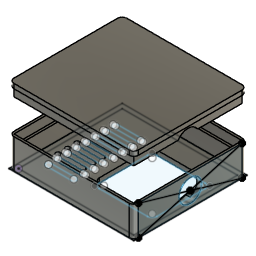
gps&speaker v2 (Autodesk Fusion 360 design; units mm, degrees)
Autodesk Fusion 360 part; units mm, degrees
sketch "Sketch1" plane through (0, 0, 0) normal (0, 0, 1) x (1, 0, 0)
  line L0 (0, 0) -> (50, 0)
  line L1 (50, 0) -> (50, 45)
  line L2 (50, 45) -> (0, 45)
  line L3 (0, 45) -> (0, 0)
  line L4 (-2, -2) -> (52, -2)
  line L5 (52, -2) -> (52, 47)
  line L6 (52, 47) -> (-2, 47)
  line L7 (-2, 47) -> (-2, -2)
  line L8 (25, 35) -> (46, 35)
  line L9 (48, 33) -> (48, 12)
  line L10 (46, 10) -> (25, 10)
  line L11 (23, 12) -> (23, 33)
  arc A0 (25, 35) -> (23, 33) centre (25, 33) ccw
  arc A1 (48, 33) -> (46, 35) centre (46, 33) ccw
  arc A2 (46, 10) -> (48, 12) centre (46, 12) ccw
  arc A3 (23, 12) -> (25, 10) centre (25, 12) ccw
  line L12 (5, 7) -> (16, 7)
  line L13 (16, 9) -> (5, 9)
  arc A4 (4, 8) -> (5, 7) centre (5, 8) ccw
  arc A5 (5, 9) -> (4, 8) centre (5, 8) ccw
  arc A6 (16, 7) -> (17, 8) centre (16, 8) ccw
  arc A7 (17, 8) -> (16, 9) centre (16, 8) ccw
  line L14 (16, 13.1429) -> (5, 13.1429)
  line L15 (5, 11.1429) -> (16, 11.1429)
  arc A8 (4, 12.1429) -> (5, 11.1429) centre (5, 12.1429) ccw
  arc A9 (5, 13.1429) -> (4, 12.1429) centre (5, 12.1429) ccw
  arc A10 (16, 11.1429) -> (17, 12.1429) centre (16, 12.1429) ccw
  arc A11 (17, 12.1429) -> (16, 13.1429) centre (16, 12.1429) ccw
  line L16 (16, 17.2857) -> (5, 17.2857)
  line L17 (5, 15.2857) -> (16, 15.2857)
  arc A12 (4, 16.2857) -> (5, 15.2857) centre (5, 16.2857) ccw
  arc A13 (5, 17.2857) -> (4, 16.2857) centre (5, 16.2857) ccw
  arc A14 (16, 15.2857) -> (17, 16.2857) centre (16, 16.2857) ccw
  arc A15 (17, 16.2857) -> (16, 17.2857) centre (16, 16.2857) ccw
  line L18 (16, 21.4286) -> (5, 21.4286)
  line L19 (5, 19.4286) -> (16, 19.4286)
  arc A16 (4, 20.4286) -> (5, 19.4286) centre (5, 20.4286) ccw
  arc A17 (5, 21.4286) -> (4, 20.4286) centre (5, 20.4286) ccw
  arc A18 (16, 19.4286) -> (17, 20.4286) centre (16, 20.4286) ccw
  arc A19 (17, 20.4286) -> (16, 21.4286) centre (16, 20.4286) ccw
  line L20 (16, 25.5714) -> (5, 25.5714)
  line L21 (5, 23.5714) -> (16, 23.5714)
  arc A20 (4, 24.5714) -> (5, 23.5714) centre (5, 24.5714) ccw
  arc A21 (5, 25.5714) -> (4, 24.5714) centre (5, 24.5714) ccw
  arc A22 (16, 23.5714) -> (17, 24.5714) centre (16, 24.5714) ccw
  arc A23 (17, 24.5714) -> (16, 25.5714) centre (16, 24.5714) ccw
  line L22 (16, 29.7143) -> (5, 29.7143)
  line L23 (5, 27.7143) -> (16, 27.7143)
  arc A24 (4, 28.7143) -> (5, 27.7143) centre (5, 28.7143) ccw
  arc A25 (5, 29.7143) -> (4, 28.7143) centre (5, 28.7143) ccw
  arc A26 (16, 27.7143) -> (17, 28.7143) centre (16, 28.7143) ccw
  arc A27 (17, 28.7143) -> (16, 29.7143) centre (16, 28.7143) ccw
  line L24 (16, 33.8571) -> (5, 33.8571)
  line L25 (5, 31.8571) -> (16, 31.8571)
  arc A28 (4, 32.8571) -> (5, 31.8571) centre (5, 32.8571) ccw
  arc A29 (5, 33.8571) -> (4, 32.8571) centre (5, 32.8571) ccw
  arc A30 (16, 31.8571) -> (17, 32.8571) centre (16, 32.8571) ccw
  arc A31 (17, 32.8571) -> (16, 33.8571) centre (16, 32.8571) ccw
  line L26 (16, 38) -> (5, 38)
  line L27 (5, 36) -> (16, 36)
  arc A32 (4, 37) -> (5, 36) centre (5, 37) ccw
  arc A33 (5, 38) -> (4, 37) centre (5, 37) ccw
  arc A34 (16, 36) -> (17, 37) centre (16, 37) ccw
  arc A35 (17, 37) -> (16, 38) centre (16, 37) ccw
  point P0 (23, 35)
  point P1 (48, 35)
  point P2 (23, 10)
  dimension "d1" = 50
  dimension "d2" = 45
  dimension "d3" = 2
  dimension "d4" = 25
  dimension "d5" = 25
  dimension "d6" = 2
  dimension "d11" = 1
  dimension "d14" = 0
  dimension "d15" = 29
  constraint horizontal L0
  constraint vertical L1
  constraint horizontal L2
  constraint vertical L3
  constraint coincident L0.start L3.end
  constraint horizontal L8
  constraint vertical L9
  constraint horizontal L10
  constraint vertical L11
  constraint coincident P0 L8
  constraint coincident P0 L11
  constraint tangent L8 A0
  constraint tangent L11 A0
  constraint coincident P1 L8
  constraint coincident P1 L9
  constraint tangent L8 A1
  constraint tangent L9 A1
  constraint equal A0 A1
  constraint tangent L9 A2
  constraint tangent L10 A2
  constraint equal A0 A2
  constraint coincident P2 L10
  constraint coincident P2 L11
  constraint tangent L10 A3
  constraint tangent L11 A3
  constraint equal A0 A3
  constraint horizontal L12
  constraint horizontal L13
  constraint tangent L12 A4
  constraint tangent L13 A5
  constraint equal A4 A5
  constraint coincident A4.start A5.end
  constraint tangent L12 A6
  constraint equal A4 A6
  constraint tangent L13 A7
  constraint equal A4 A7
  constraint coincident A6.end A7.start
  measures "d1" distance of L0.start L0.end
  measures "d2" distance of L0.start L2.end
  measures "d4" distance of P0 P1
  measures "d5" distance of P0 P2
  measures "d6" radius of A0
  measures "d11" radius of A4
extrude "Extrude1" add sketch "Sketch1" along normal blind 15 contours L4 L5 L6 L7 makes body 1
extrude "Extrude2" add sketch "Sketch1" along normal blind 2 contours L0 L1 L2 L3 | L12 L13 A4 A5 A6 A7 | L14 L15 A8 A9 A10 A11 | L16 L17 A12 A13 A14 A15 | L18 L19 A16 A17 A18 A19 | L20 L21 A20 A21 A22 A23 | L22 L23 A24 A25 A26 A27 | L24 L25 A28 A29 A30 A31 | L26 L27 A32 A33 A34 A35 bodies 1
extrude "Extrude3" cut sketch "Sketch1" along normal blind 3 contours L12 L13 A4 A5 A6 A7 | L14 L15 A8 A9 A10 A11 | L16 L17 A12 A13 A14 A15 | L18 L19 A16 A17 A18 A19 | L20 L21 A20 A21 A22 A23 | L22 L23 A24 A25 A26 A27 | L24 L25 A28 A29 A30 A31 | L26 L27 A32 A33 A34 A35 bodies 1
sketch "Sketch2" plane through (0, 0, 0) normal (0, 1, 0) x (-1, 0, 0)
  line L0 (-50, 2) -> (0, 2)
  line L1 (0, 2) -> (0, 15)
  line L2 (0, 15) -> (-50, 15)
  line L3 (-50, 15) -> (-50, 2)
  line L4 (-50, 15) -> (0, 15)
  line L5 (0, 15) -> (0, 13)
  line L6 (0, 13) -> (-50, 13)
  line L7 (-50, 13) -> (-50, 15)
  constraint horizontal L4
  constraint vertical L5
  constraint horizontal L6
  constraint vertical L7
  constraint coincident L1 L5.end
  constraint coincident L2.end L3.start
extrude "Extrude4" add sketch "Sketch2" along normal blind 45 contours L1 L2 L3 L4 L5 L6 L7 bodies 1
split "Split1" by plane through (0, 0, 13) normal (0, 0, -1) bodies 1 makes body 2 at (22.0474, 1.0034, 0)
move_body "Move1" bodies 1 to x (1, 0, 0) y (0, 1, 0) z (0, 0, 1) at (0, 0, 17)
sketch "Sketch3" plane through (0, 0, 13) normal (0, 0, 1) x (-1, 0, 0)
  line L0 (-52, -47) -> (2, -47)
  line L1 (2, -47) -> (2, 2)
  line L2 (2, 2) -> (-52, 2)
  line L3 (-52, 2) -> (-52, -47)
  line L4 (-50, 0) -> (0, 0)
  line L5 (0, 0) -> (0, -45)
  line L6 (0, -45) -> (-50, -45)
  line L7 (-50, -45) -> (-50, 0)
  line L8 (-51, 1) -> (1, 1)
  line L9 (1, 1) -> (1, -46)
  line L10 (1, -46) -> (-51, -46)
  line L11 (-51, -46) -> (-51, 1)
  dimension "d20" = -1
extrude "Extrude5" cut sketch "Sketch3" against normal blind 4 contours L8 L9 L10 L11 bodies 2
extrude "Extrude6" add 1 faces at (33.3333, -0.6667, 9) along direction (0, 0, 1) blind 17 and the other way blind -21 on bodies 2 bodies 2 1
fillet "Fillet1" radius 2 8 edges at (52, 47, 31) (52, -2, 31) (-2, -2, 31) (-2, 47, 31) (-2, 47, 6.5) (-2, -2, 6.5) (52, -2, 6.5) (52, 47, 6.5) on bodies 1 2
sketch "Sketch4" plane through (52, 0, 0) normal (1, 0, 0) x (0, 1, 0)
  line L0 (45, 0) -> (45, 13)
  line L1 (45, 13) -> (0, 13)
  line L2 (0, 13) -> (0, 0)
  line L3 (0, 0) -> (45, 0)
  line L4 (0, 13) -> (45, 0)
  line L5 (45, 13) -> (0, 0)
  circle A0 centre (22.5, 6.5) radius 4.8836
  constraint coincident L1.end L2.start
  constraint coincident L0.start L3.end
  constraint coincident L0.end L1.start
  constraint coincident L2.end L3.start
  constraint midpoint L5 A0.centre
extrude "Extrude7" cut sketch "Sketch4" against normal blind 5 contours L4 L5 A0 | L4 L5 A0 | L4 L5 A0 | L4 L5 A0 bodies 2
move_body "Move2" bodies 1 to x (1, 0, 0) y (0, 1, 0) z (0, 0, 1) at (0, 0, -17)
extrude "Extrude8" cut sketch "Sketch4" against normal blind 6 contours L4 L5 A0 | L4 L5 A0 | L4 L5 A0 | L4 L5 A0 bodies 1
move_body "Move3" bodies 1 to x (1, 0, 0) y (0, 1, 0) z (0, 0, 1) at (0, 0, 18)
